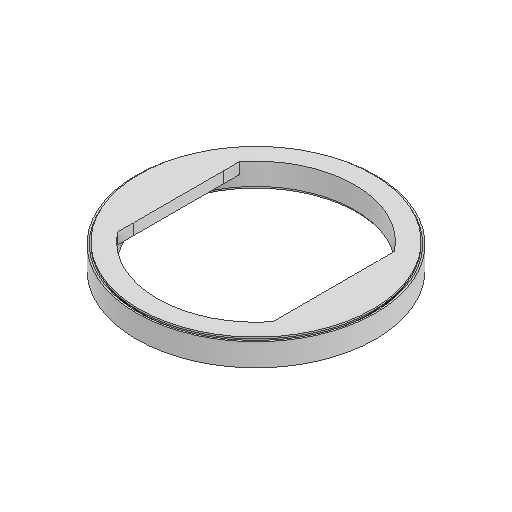
# Autodesk Inventor part: roofparts_support_upper
Saved by Autodesk Inventor 2022.6 (Build 266554000, 554)
## iProperties
Created: 2024-10-26
Part Number: roofparts_support_upper
Material: 一般
Document SubType Name: Modeling
Designer: acbaf
Density: 1 g/cm^3
Appearance: 既定
Author: acbaf
## iProperties of the stored document roofparts_support_upper_3D プリント.ipt
Created: 2024-10-26
Part Number: roofparts_support_upper_3D プリント
Material: 一般
Document SubType Name: Modeling
Designer: acbaf
Density: 1 g/cm^3
Appearance: 既定
Author: acbaf
Autodesk Inventor part; units mm, degrees
ref_plane "YZ Plane" through (0, 0, 0) normal (1, 0, 0) x (0, 1, 0)
ref_plane "XZ Plane" through (0, 0, 0) normal (0, 1, 0) x (-1, 0, 0)
ref_plane "XY Plane" through (0, 0, 0) normal (0, 0, 1) x (1, 0, 0)
sketch "スケッチ1" plane through (0, 0, 0) normal (0, 1, 0) x (-1, 0, 0)
  circle A0 centre (0, 0) radius 49.5
  circle A1 centre (0, 0) radius 60
  circle A2 centre (0, 0) radius 47.5
  circle A3 centre (0, 0) radius 45
  line L0 (42.8856, 24.7199) -> (-42.8508, -24.7801)
  line L1 (0, -84) -> (0, 84) projected
  line L2 (-42.8856, 24.7199) -> (42.8508, -24.7801)
  line L3 (38.9537, -22.5301) -> (38.9885, 22.4699)
  line L4 (-38.9537, -22.5301) -> (-38.9885, 22.4699)
  point P0 (38.9885, 22.4699)
  point P1 (38.9537, -22.5301)
  point P2 (-38.9885, 22.4699)
  point P3 (38.9537, -22.5301)
  dimension "d0" = 99
  dimension "d1" = 120
  dimension "d4" = 95
  dimension "d7" = 90
  dimension "d8" = 60
  constraints: 8 end point, 6 point on circle, 4 centre point, 4 coincident, 4 point on line, 2 symmetric about line
  measures "d0" diameter of A0
  measures "d1" diameter of A1
  measures "d4" diameter of A2
  measures "d7" diameter of A3
  measures "d8" angle of L1 L0
extrude "押し出し1" add sketch "スケッチ1" along normal blind 6.8 contours A0 L1 A1 | A0 L1 A1
extrude "押し出し2" add sketch "スケッチ1" along normal blind 6 from surface at 6.8 separate body contours A0 L2 A2 L0 | A2 L2 A3 L0 | L2 A2 L0 A0 | A3 L3 | L2 A3 L0 A2 | L4 A3
sketch "スケッチ5" plane through (0, 0, 0) normal (0, 0, 1) x (1, 0, 0)
  line L0 (49.5, 6.8) -> (49.5, 12.8) projected
  line L1 (60, 0) -> (60, 6.8) projected
  line L2 (60, 6.8) -> (-60, 6.8) projected
  line L3 (60, 0) -> (-60, 0) projected
  line L4 (42.8508, 12.8) -> (42.8856, 12.8) projected
  line L5 (42.8856, 12.8) -> (42.8856, 6.8) projected
  line L6 (42.8508, 6.8) -> (42.8856, 6.8) projected
  line L7 (42.8508, 6.8) -> (42.8508, 12.8) projected
  line L8 (42.8508, 12.8) -> (49.5, 12.8) projected
  line L9 (49.5, 12.8) -> (60, 12.8)
  line L10 (60, 6.8) -> (60, 12.8)
  line L11 (0, -2.56) -> (0, 15.36) projected
  line L12 (0, 46) -> (10, 46)
  line L13 (10, -13.316) -> (10, 46)
  line L14 (10, 46) -> (0, 46)
  line L15 (0, 46) -> (0, 36)
  line L16 (0, 36) -> (10, 36)
  line L17 (10, 36) -> (10, 46)
  line L18 (0, 36) -> (10, 46)
  circle A0 centre (5, 41) radius 3
  circle A1 centre (5, 41) radius 3.1
  circle A2 centre (5, 41) radius 3.3
  line L19 (0.4243, 36) -> (10.4879, 46.0636)
  line L20 (-0.4243, 36) -> (9.8636, 46.2879)
  line L21 (10, 44.3757) -> (8.8, 44.3757)
  line L22 (-2.5994, 0) -> (14.1115, 0)
  line L23 (0, 46) -> (10, 46)
  line L24 (8.3757, 46) -> (8.3757, 44.8)
  line L25 (0, 46) -> (-1.5, 46)
  line L26 (-1.5, 46) -> (-1.5, 36)
  line L27 (-1.5, 36) -> (0, 36)
  line L28 (0, 36) -> (0, 46)
  line L29 (-49.5, 0) -> (49.5, 0) projected
  line L30 (60, 12.8) -> (49.5, 0) construction
  line L31 (60, 0) -> (-60, 0) projected
  line L32 (49.5, 12.8) -> (60, 0) construction
  circle A3 centre (54.75, 6.4) radius 3 construction
  circle A4 centre (54.75, 6.4) radius 3.1
  circle A5 centre (54.75, 6.4) radius 3.3
  line L33 (60, 12.327) -> (49.888, 0)
  line L34 (59.612, 12.8) -> (49.112, 0)
  line L35 (60, 12.4) -> (42.8508, 12.4)
  line L36 (58.6276, 12.4) -> (58.6276, 11.6)
  line L37 (60, 11.3517) -> (59.2, 11.3517)
  line L38 (49.5, 6.8) -> (49.5, 0.473)
  line L39 (50.5443, 0.8) -> (50.5443, 0)
  line L40 (42.8508, 12.8) -> (38.4142, 12.8)
  line L41 (38.4142, 12.8) -> (38.4142, 12.4)
  line L42 (38.4142, 12.4) -> (42.8508, 12.4)
  line L43 (42.8508, 12.4) -> (42.8508, 12.8)
  line L44 (42.8306, 12.4) -> (42.8856, 12.4)
  line L45 (50.3, 1.4483) -> (49.5, 1.4483)
  point P0 (0, 0)
  point P1 (0, 0)
  point P2 (3.0304, 38.6061)
  point P3 (7.3939, 42.9696)
  point P4 (0, 36.4243)
  point P5 (2.4641, 38.8883)
  point P6 (7.1117, 43.5359)
  point P7 (56.6023, 9.1311)
  point P8 (52.4338, 4.0494)
  point P9 (56.9388, 8.5952)
  point P10 (53.0251, 3.8242)
  dimension "d26" = 10
  dimension "d27" = 10
  dimension "d28" = 6
  dimension "d29" = 5
  dimension "d30" = 5
  dimension "d31" = 0.1
  dimension "d32" = 0.3
  dimension "d33" = 0.3
  dimension "d34" = 0.3
  dimension "d35" = 1.2
  dimension "d36" = 1.2
  dimension "d37" = 1.5
  dimension "d38" = 10
  dimension "d39" = 6
  dimension "d40" = 0.1
  dimension "d41" = 0.3
  dimension "d42" = 0.3
  dimension "d43" = 0.3
  dimension "d46" = 0.4
  dimension "d47" = 0.8
  dimension "d48" = 0.8
  dimension "d49" = 0.8
  dimension "d50" = 0.4
  dimension "d53" = 0.8
  constraints: 68 end point, 21 point on line, 11 parallel, 7 perpendicular, 6 centre point, 5 horizontal, 3 midpoint, 3 vertical, 4 other
  measures "d26" distance of L16.end L15.end
  measures "d27" distance of L15.end L14.end
  measures "d28" diameter of A0
  measures "d29" distance from line of A0.centre L13
  measures "d30" distance from line of L16 A0.centre
  measures "d31" radial gap between concentric circles of A0 A1
  measures "d32" radial gap between concentric circles of A0 A2
  measures "d33" distance between parallel lines of L18 L19
  measures "d34" distance between parallel lines of L18 L20
  measures "d35" distance of L21.start L21.end
  measures "d36" distance of L24.start L24.end
  measures "d37" distance of L27.end L26.end
  measures "d38" distance of L26.end L25.end
  measures "d39" diameter of A3
  measures "d40" radial gap between concentric circles of A3 A4
  measures "d41" radial gap between concentric circles of A3 A5
  measures "d42" distance between parallel lines of L34 L30
  measures "d43" distance between parallel lines of L30 L33
  measures "d46" distance between parallel lines of L8 L35
  measures "d47" distance of L36.start L36.end
  measures "d48" distance of L37.start L37.end
  measures "d49" distance of L39.start L39.end
  measures "d50" distance of L41.end L40.end
  measures "d53" distance of L45.start L45.end
revolve "回転5" add sketch "スケッチ5" angle 360 mid plane about axis through (0, -10, 0) along (0, 1, 0) picked at (54.2272, 9.5719) picked at (52.7365, 7.026) picked at (56.9325, 8.6926) picked at (55.5437, 7.5253) picked at (57.683, 7.7179) picked at (56.9846, 7.0196) bodies 1 contours L0 L35 L36 L34 A5 L2 | L0 L9 L34 L35 | A5 L34 A4 L2 | L35 L34 L36 | A4 L34 L2 | L34 L35 L10 L33 A5 | A5 L33 A4 L34 | L9 L10 L35 L34 | L34 A4 L33 L2 | L33 L37 L10 L2 A5 | A5 L2 A4 L33 | L33 A4 L2 | L33 L10 L37
revolve "回転6" cut sketch "スケッチ5" angle 360 about axis through (0, -10, 0) along (0, -1, 0) bodies 1 2 contours L35 L5 L8 L0 | L0 L9 L34 L35 | A5 L34 A4 L2 | L2 A4 L34 A5 | L45 L34 L38 | L35 L34 L36 | L35 L7 L4 L5 | A4 L34 L2 | L2 L34 A4 | L34 L35 L10 L33 A5 | A5 L33 A4 L34 | L34 A4 L33 A5 | A5 L33 L3 L34 | L9 L10 L35 L34 | L42 L41 L40 L7 | L34 A4 L33 L2 | L2 L33 A4 L34 | L33 L37 L10 L2 A5 | A5 L2 A4 L33 | L33 A4 L2 A5 | A5 L2 L1 L3 L39 L33 | L33 A4 L2 | L2 A4 L33 | L33 L10 L37 | L39 L3 L33
combine bodies "結合2" operation type add bodies to combine 1 2
revolve "回転7" add sketch "スケッチ5" angle 360 about axis through (0, -10, 0) along (0, -1, 0) separate body contours L33 L37 L10 L2 A5 | A5 L2 A4 L33 | L33 A4 L2 A5 | A5 L2 L1 L3 L39 L33
sketch "スケッチ6" plane through (0, 12.4, 0) normal (0, 1, 0) x (1, 0, 0)
  arc A0 (42.8508, 24.7801) -> (-42.8508, 24.7801) centre (0, 0) ccw projected
  line L0 (38.9537, 22.5301) -> (42.8508, 24.7801) projected
  line L1 (38.9885, -22.4699) -> (38.9537, 22.5301) projected
  line L2 (42.8856, -24.7199) -> (38.9885, -22.4699) projected
  arc A1 (-42.8856, -24.7199) -> (42.8856, -24.7199) centre (0, 0) ccw projected
  line L3 (-38.9885, -22.4699) -> (-42.8856, -24.7199) projected
  line L4 (-38.9537, 22.5301) -> (-38.9885, -22.4699) projected
  line L5 (-42.8508, 24.7801) -> (-38.9537, 22.5301) projected
  circle A2 centre (0, 0) radius 58.6276 projected
  line L6 (38.9537, 22.5301) -> (38.9537, 30.5427)
  circle A3 centre (0, 0) radius 49.5 projected
  line L7 (38.9885, -22.4699) -> (38.9885, -30.4983)
  line L8 (0, -0.9078) -> (0, -8.1069) construction
  line L9 (-38.9537, 22.5301) -> (-38.9537, 30.5427)
  line L10 (-38.9885, -22.4699) -> (-38.9885, -30.4983)
  constraints: 10 end point, 3 vertical, 2 point on circle, 2 symmetric about line, 1 point on line
extrude "押し出し3" add sketch "スケッチ6" against normal blind 5.6 contours L0 L6 A0 | L9 L5 A0 | L2 A1 L7 | L3 L10 A1 bodies 1
sketch "スケッチ7" plane through (38.9885, 6.8, 22.4699) normal (0, -1, 0) x (1, 0, 0)
  line L0 (0, 0) -> (-0.0348, -45) projected
  line L1 (-0.0348, -45) -> (-0.0348, -53.0126) projected
  arc A0 (-0.0348, -53.0126) -> (0, 8.0284) centre (-38.9885, -22.4699) ccw projected
  line L2 (0, 8.0284) -> (0, 0) projected
  line L3 (-77.9423, -45) -> (-77.9771, 0) projected
  line L4 (-77.9771, 0) -> (-77.9771, 8.0284) projected
  arc A1 (-77.9771, 8.0284) -> (-77.9423, -53.0126) centre (-38.9885, -22.4699) ccw projected
  line L5 (-77.9423, -53.0126) -> (-77.9423, -45) projected
extrude "押し出し4" add sketch "スケッチ7" along normal blind 1 separate body contours L2 A0 L1 L0
